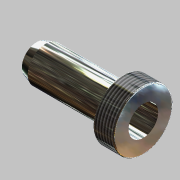
# Autodesk Inventor part: YTP-AP-E12-R1.0
Saved by Autodesk Inventor 2020.4 (Build 244396010, 396A)
## iProperties
RuleStatus: InUse
AfterDocNew0: iPropertyEnforcement
BeforeDocSave0: Materialprüfung
Created: 2021-08-29
Part Number: YTP-AP-E12-R1.0
Material: Allgemein
Document SubType Name: Modeling
Designer: Uwe Wieser
Mass: 0.334995 g
Surface Area: 7.76629 cm^2
Volume: 0.334995 cm^3
Density: 1 g/cm^3
Appearance: Chrom - poliert
Project: Airbrush
Description: Federaufnahme
Werkstoff: 1.4301
Author: Uwe Wieser
Autodesk Inventor part; units mm, degrees
ref_plane "YZ Plane" through (0, 0, 0) normal (1, 0, 0) x (0, 1, 0)
ref_plane "XZ Plane" through (0, 0, 0) normal (0, 1, 0) x (-1, 0, 0)
ref_plane "XY Plane" through (0, 0, 0) normal (0, 0, 1) x (1, 0, 0)
sketch "Skizze1" plane through (0, 0, 0) normal (0, 0, 1) x (1, 0, 0)
  line L0 (-16.5, 2.5) -> (0, 2.5)
  line L1 (0, 5) -> (-3.5, 5)
  line L2 (0, 5) -> (0, 2.5)
  line L3 (-3.5, 5) -> (-3.5, 3)
  line L4 (-3.5, 3) -> (-16.5, 3)
  line L5 (-18, 2.5) -> (-16.5, 3)
  line L6 (-16.5, 2) -> (-18, 2)
  line L7 (-16.5, 2) -> (-16.5, 2.5)
  line L8 (-18, 2.5) -> (-18, 2)
  line L9 (0, 1.4) -> (0, 5.6) projected
  line L10 (-21.6, 0) -> (3.6, 0) projected
  dimension "d0" = 5
  dimension "d1" = 10
  dimension "d2" = 6
  dimension "d3" = 1.5
  dimension "d4" = 4
  dimension "d5" = 18
  dimension "d6" = 3.5
  dimension "d7" = 161.565
  constraints: 18 end point, 2 parallel, 2 point on line
  measures "d0" diameter of L0 L10
  measures "d1" diameter of L1 L10
  measures "d2" diameter of L4 L10
  measures "d3" distance of L6.start L6.end
  measures "d4" diameter of L6 L10
  measures "d5" distance between parallel lines of L9 L8
  measures "d6" distance of L1.start L1.end
  measures "d7" angle of L4 L5
revolve "Umdrehung1" add sketch "Skizze1" angle 360 about axis through (-10, 0, 0) along (1, 0, 0)
thread "Gewinde1" size "M10x0.5" class "6g" standard "ISO Metric profile" full length
fillet "Rundung1" radius 0.2 3 edges at (-3.5, -3, 0) (-3.5, -5, 0) (0, -5, 0)
